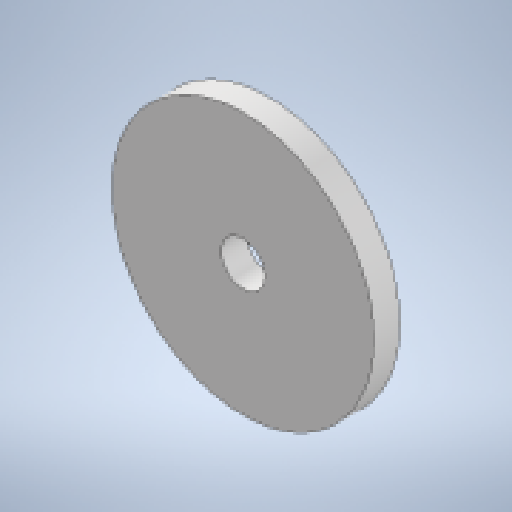
# Autodesk Inventor part: Pad_2
Saved by Autodesk Inventor 2023 (Build 270158000, 158)
## iProperties
Created: 2022-04-08
Part Number: Pad_2
Material: 一般
Document SubType Name: Modeling
Designer: device
Mass: 3.31193 g
Surface Area: 28.3957 cm^2
Volume: 3.31193 cm^3
Density: 1 g/cm^3
Appearance: 預設
Author: device
Autodesk Inventor part; units mm, degrees
ref_plane "YZ Plane" through (0, 0, 0) normal (1, 0, 0) x (0, 1, 0)
ref_plane "XZ Plane" through (0, 0, 0) normal (0, 1, 0) x (-1, 0, 0)
ref_plane "XY Plane" through (0, 0, 0) normal (0, 0, 1) x (1, 0, 0)
sketch "草圖1" plane through (0, 0, 0) normal (0, 0, 1) x (1, 0, 0)
  circle A0 centre (0, 0) radius 2.5
  circle A1 centre (0, 0) radius 15
  dimension "d0" = 5
  dimension "d1" = 30
  constraints: 2 centre point, 2 coincident
  measures "d0" diameter of A0
  measures "d1" diameter of A1
extrude "擠出1" add sketch "草圖1" along normal mid plane 3
sketch "草圖2" plane through (0, 0, -1.5) normal (0, 0, -1) x (-1, 0, 0)
  circle A0 centre (0, 0) radius 15 projected
  circle A1 centre (0, 0) radius 2.5 construction
  line L0 (0, 15) -> (-15, 15)
  line L1 (-15, 15) -> (-15, -15)
  line L2 (-15, -15) -> (0, -15)
  line L3 (0, -15) -> (0, 15) construction
  circle A2 centre (0, 0) radius 15 projected
  point P0 (0, -15)
  point P1 (-15, 0)
  constraints: 8 end point, 2 parallel, 1 horizontal, 1 perpendicular, 1 point on circle, 1 vertical, 2 other
extrude "擠出2" add sketch "草圖2" against normal blind 3 contours A0 L1 L0 | L2 L1 A0
sketch "草圖3" plane through (0, 0, -1.5) normal (0, 0, -1) x (-1, 0, 0)
  arc A0 (0, -15) -> (0, 15) centre (0, 0) ccw projected
  line L0 (0, 15) -> (-15, 15) projected
  line L1 (-15, 15) -> (-15, -15) projected
  line L2 (-15, -15) -> (0, -15) projected
  circle A1 centre (0, 0) radius 2.5 projected
  line L3 (-15, 15) -> (0, 15) projected
  line L4 (-12, 18) -> (-15, 18)
  line L5 (-15, 18) -> (-15, -18)
  line L6 (-15, -18) -> (-12, -18)
  line L7 (-12, -18) -> (-12, 18)
  point P0 (-15, 0)
  dimension "d13" = 36
  dimension "d14" = 3
  constraints: 8 end point, 2 midpoint, 2 parallel, 1 horizontal, 1 perpendicular
  measures "d13" distance of L4.end L5.end
  measures "d14" distance of L4.start L4.end
extrude "擠出3" add sketch "草圖3" along normal blind 17.5 contours L7 L6 L5 L2 | L2 L1 L0 L7 | L0 L5 L4 L7
sketch "草圖5" plane through (0, 0, -19) normal (0, 0, -1) x (-1, 0, 0)
  line L0 (-12, -18) -> (-12, 18) projected
  line L1 (-12, 18) -> (-15, 18) projected
  line L2 (-15, 18) -> (-15, -18) projected
  line L3 (-15, -18) -> (-12, -18) projected
  line L4 (-15, 12) -> (-12, 12)
  line L5 (-12, 12) -> (-12, -12)
  line L6 (-12, -12) -> (-15, -12)
  line L7 (-15, -12) -> (-15, 12)
  point P0 (0, 0)
  point P1 (-15, 0)
  point P2 (-13.5, -12)
  point P3 (-13.5, 12)
  dimension "d15" = 24
  constraints: 8 end point, 4 midpoint, 2 parallel, 2 point on line, 1 horizontal, 1 perpendicular
  measures "d15" distance of point (-13.5, -12) point (-13.5, 12)
extrude "擠出5" cut sketch "草圖5" against normal blind 12.5 contours L6 L2 L4 L0
sketch "草圖6" plane through (12, -18, -1.5) normal (-1, 0, 0) x (0, 0, 1)
  line L0 (-17.5, 30) -> (-5, 30) construction
  line L1 (-5, 30) -> (-5, 6) construction
  line L2 (-5, 6) -> (-17.5, 6) construction
  line L3 (-17.5, 0) -> (-17.5, 6) construction
  line L4 (0, 0) -> (-17.5, 0) construction
  line L5 (0, 0) -> (0, 3) construction
  line L6 (0, 33) -> (0, 3) construction
  line L7 (0, 33) -> (0, 36) construction
  line L8 (0, 36) -> (-17.5, 36) construction
  line L9 (-17.5, 30) -> (-17.5, 36) construction
  line L10 (-11.25, 36) -> (-11.25, 0) construction
  line L11 (0, 0) -> (-17.5, 0) construction
  circle A0 centre (-11.25, 32.5) radius 1.25
  circle A1 centre (-11.25, 3.5) radius 1.25
  line L12 (-11.25, 18) -> (-8.75, 18) construction
  point P0 (1.5, 18)
  point P1 (-11.25, 30)
  dimension "d18" = 2.5
  dimension "d19" = 29
  constraints: 5 point on line, 4 end point, 2 centre point, 2 midpoint, 1 equal radius, 1 horizontal, 1 perpendicular, 1 symmetric about line
  measures "d18" diameter of A0
  measures "d19" distance of A1.centre A0.centre
extrude "擠出6" cut sketch "草圖6" against normal up to surface (3 mm away)
